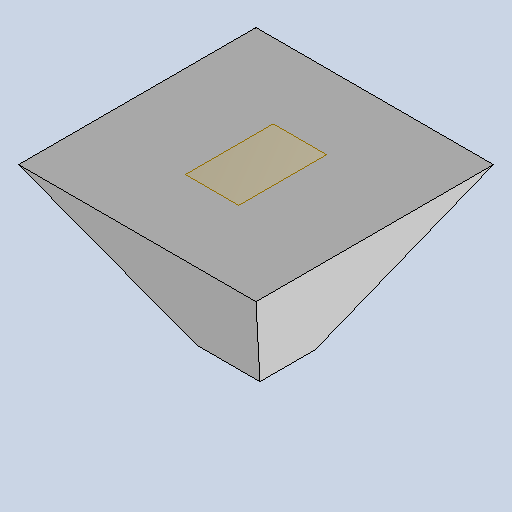
# Autodesk Inventor part: NDM-VOS dummy2
Saved by Autodesk Inventor 2025 (Build 290162010, 162A)
## iProperties
Created: 2024-07-24
Part Number: NDM-VOS dummy2
Material: Water
Document SubType Name: Modeling
Designer: admin
Mass: 1.00163e+06 g
Surface Area: 67468.3 cm^2
Volume: 1.00333e+06 cm^3
Density: 0.9983 g/cm^3
Appearance: Default
Author: admin
Autodesk Inventor part; units mm, degrees
ref_plane "YZ Plane" through (0, 0, 0) normal (1, 0, 0) x (0, 1, 0)
ref_plane "XZ Plane" through (0, 0, 0) normal (0, 1, 0) x (-1, 0, 0)
sketch "Sketch2" plane through (0, 0, 0) normal (0, 0, 1) x (1, 0, 0)
  line L0 (200, -175) -> (-200, -175)
  line L1 (-200, -175) -> (-200, 175)
  line L2 (-200, 175) -> (200, 175)
  line L3 (200, 175) -> (200, -175)
  line L4 (200, -175) -> (-200, 175) construction
  line L5 (-200, -175) -> (200, 175) construction
  point P0 (0, 0)
  point P1 (0, 0)
  dimension "d9" = 350
  dimension "d16" = 400
  constraints: 12 end point, 2 coincident, 2 midpoint, 2 parallel, 1 horizontal, 1 perpendicular
  measures "d9" distance of L0.end L1.end
  measures "d16" distance of L0.start L0.end
ref_plane "Work Plane1" through (0, 0, 1000) normal (0, 0, 1) x (1, 0, 0)
sketch "Sketch3" plane through (0, 0, 1000) normal (0, 0, 1) x (1, 0, 0)
  line L0 (750, 750) -> (-750, 750)
  line L1 (-750, 750) -> (-750, -750)
  line L2 (-750, -750) -> (750, -750)
  line L3 (750, -750) -> (750, 750)
  line L4 (750, 750) -> (-750, -750) construction
  line L5 (-750, 750) -> (750, -750) construction
  point P0 (0, 0)
  point P1 (0, 0)
  dimension "d11" = 1500
  dimension "d17" = 1500
  constraints: 12 end point, 2 midpoint, 2 parallel, 1 coincident, 1 horizontal, 1 perpendicular
  measures "d11" distance of L0.end L1.end
  measures "d17" distance of L1.end L2.end
loft "Loft1" add profiles "Sketch3", "Sketch2"
equation "\"d9\" = Конус_дно_длина"
equation "\"d16\" = Конус_дно_ширина"
equation "\"d11\" = Конус_Базовая_длина"
equation "\"d17\" = Конус_Базовая_ширина"
equation "\"Конус_дно_длина\" = 350"
equation "\"Конус_дно_ширина\" = 400"
equation "\"Конус_Базовая_длина\" = 1500"
equation "\"Конус_Базовая_ширина\" = 1500"
body "Solid2"
